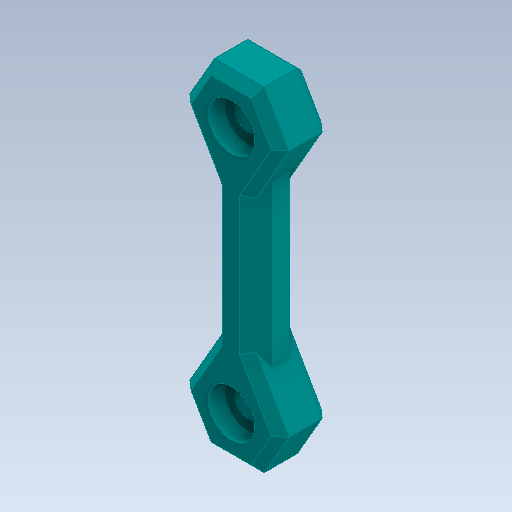
# Autodesk Inventor part: Tibia Joint
Saved by Autodesk Inventor 2020 (Build 240168000, 168)
## iProperties
Created: 2020-09-14
Part Number: Tibia Joint
Material: Generic
Document SubType Name: Modeling
Designer: Turing
Density: 1 g/cm^3
Appearance: Turquoise
Mass: 1.39468 g
Surface Area: 11.9511 cm^2
Volume: 1.39468 cm^3
Author: Turing
Autodesk Inventor part; units mm, degrees
ref_plane "YZ Plane" through (0, 0, 0) normal (1, 0, 0) x (0, 1, 0)
ref_plane "XZ Plane" through (0, 0, 0) normal (0, 1, 0) x (-1, 0, 0)
ref_plane "XY Plane" through (0, 0, 0) normal (0, 0, 1) x (1, 0, 0)
sketch "Sketch1" plane through (0, 0, 0) normal (0, 0, 1) x (1, 0, 0)
  circle A0 centre (0, 0) radius 1.55
  circle A1 centre (0, 0) radius 3
  line L0 (0, 0) -> (0, 30)
  circle A2 centre (0, 30) radius 1.55
  circle A3 centre (0, 30) radius 3
  line L1 (3, 0) -> (3, 30)
  line L2 (-3, 0) -> (-3, 30)
  line L3 (6, 30) -> (3, 24.8038)
  line L4 (3, 24.8038) -> (-3, 24.8038)
  line L5 (-3, 24.8038) -> (-6, 30)
  line L6 (-6, 30) -> (-3, 35.1962)
  line L7 (-3, 35.1962) -> (3, 35.1962)
  line L8 (3, 35.1962) -> (6, 30)
  line L9 (6, 0) -> (3, -5.1962)
  line L10 (3, -5.1962) -> (-3, -5.1962)
  line L11 (-3, -5.1962) -> (-6, 0)
  line L12 (-6, 0) -> (-3, 5.1962)
  line L13 (-3, 5.1962) -> (3, 5.1962)
  line L14 (3, 5.1962) -> (6, 0)
  point P0 (3, 24.8038)
  point P1 (-3, 24.8038)
  dimension "d0" = 3.1
  dimension "d1" = 6
  dimension "d2" = 30
  dimension "d3" = 3.1
  dimension "d4" = 6
  dimension "d5" = 30
  dimension "d6" = 3
  dimension "d7" = 6
  dimension "d8" = 6
  constraints: 30 end point, 6 coincident, 4 centre point, 4 point on circle, 2 parallel, 1 horizontal, 1 tangent, 1 vertical, 26 other
  measures "d0" diameter of A0
  measures "d1" diameter of A1
  measures "d2" distance of L0.start L0.end
  measures "d3" diameter of A2
  measures "d4" diameter of A3
  measures "d5" distance of L1.start L1.end
  measures "d6" distance from line of L2 A3.centre
  measures "d7" distance of L0.end L3.start
  measures "d8" distance of L9.start point (0, 0)
extrude "Extrusion1" add sketch "Sketch1" along normal blind 3
sketch "Sketch2" plane through (0, 0, 3) normal (0, 0, 1) x (1, 0, 0)
  circle A0 centre (0, 0) radius 2.8
  line L0 (3, 5.1962) -> (3, 24.8038) projected
  line L1 (3, 24.8038) -> (6, 30) projected
  line L2 (6, 30) -> (3, 35.1962) projected
  line L3 (3, 35.1962) -> (-3, 35.1962) projected
  line L4 (-3, 35.1962) -> (-6, 30) projected
  line L5 (-6, 30) -> (-3, 24.8038) projected
  line L6 (-3, 24.8038) -> (-3, 5.1962) projected
  line L7 (-3, 5.1962) -> (-6, 0) projected
  line L8 (-6, 0) -> (-3, -5.1962) projected
  line L9 (-3, -5.1962) -> (3, -5.1962) projected
  line L10 (3, -5.1962) -> (6, 0) projected
  line L11 (6, 0) -> (3, 5.1962) projected
  circle A1 centre (0, 30) radius 1.55 projected
  circle A2 centre (0, 0) radius 1.55 projected
  circle A3 centre (0, 30) radius 2.8
  dimension "d11" = 5.6
  dimension "d12" = 5.6
  constraints: 2 centre point, 2 coincident
  measures "d11" diameter of A0
  measures "d12" diameter of A3
extrude "Extrusion2" cut sketch "Sketch2" against normal blind 2 contours A0 | A3
chamfer "Chamfer1" distance 2 angle 45 2 edges at (-3, 15, 3) (3, 15, 3)
chamfer "Chamfer2" distance 1 angle 45 10 edges at (-4.5, 2.5981, 3) (-4.5, -2.5981, 3) (0, -5.1962, 3) (4.5, -2.5981, 3) (4.5, 2.5981, 3) (4.5, 27.4019, 3) (-4.5, 27.4019, 3) (4.5, 32.5981, 3) (0, 35.1962, 3) (-4.5, 32.5981, 3)
mirror "Mirror1" about plane through (0, 15, 0) normal (0, 0, -1)
equation "\"d0\" = d3"
equation "\"d1\" = d4"
equation "\"d5\" = d2"
equation "\"d8\" = d7"
equation "\"d12\" = d11"
body "Solid1"
